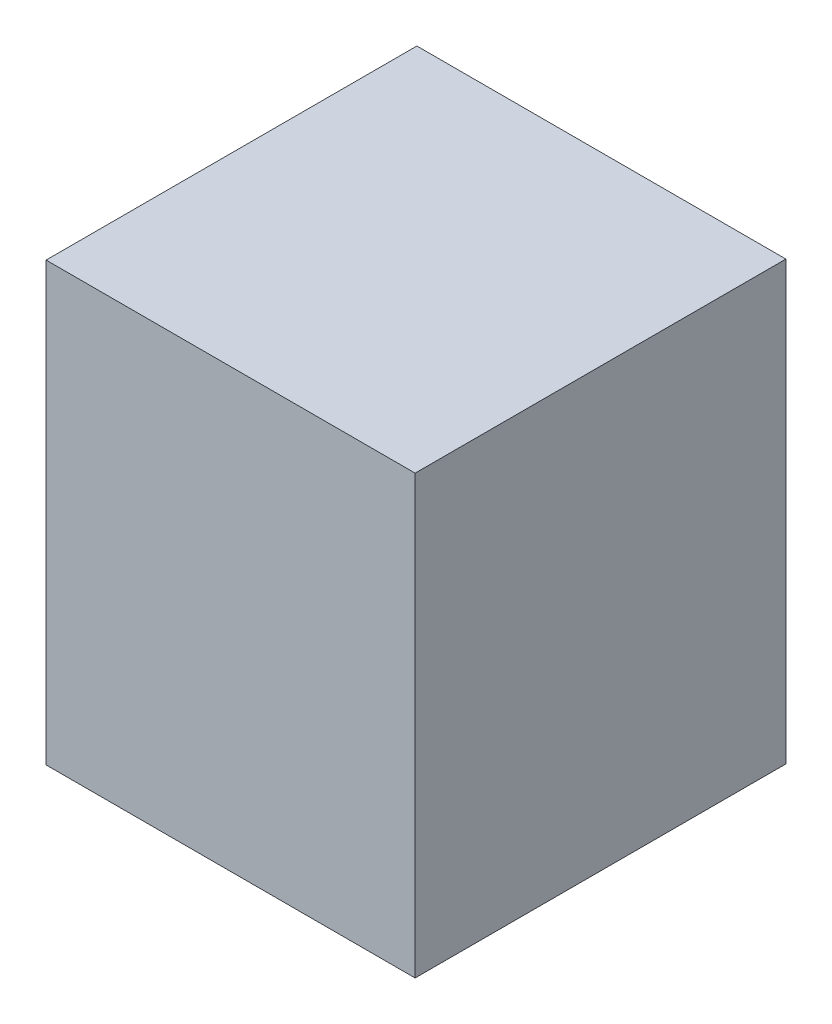
# Autodesk Inventor part: 3d printing workspace
Saved by Autodesk Inventor 2021 (Build 250183000, 183)
## iProperties
Created: 2021-11-22
Part Number: 3d printing workspace
Material: Generic
Document SubType Name: Sheet Metal
Designer: techv
Mass: 11183 g
Surface Area: 3009.64 cm^2
Volume: 11183 cm^3
Density: 1 g/cm^3
Sheet Metal Rule: Default
Appearance: Default
Author: techv
Autodesk Inventor part; units mm, degrees
ref_plane "YZ Plane" through (0, 0, 0) normal (1, 0, 0) x (0, 1, 0)
ref_plane "XZ Plane" through (0, 0, 0) normal (0, 1, 0) x (-1, 0, 0)
ref_plane "XY Plane" through (0, 0, 0) normal (0, 0, 1) x (1, 0, 0)
sketch "Sketch1" plane through (0, 0, 0) normal (0, 1, 0) x (-1, 0, 0)
  line L0 (-105.5, 106) -> (105.5, 106)
  line L1 (105.5, 106) -> (105.5, -106)
  line L2 (105.5, -106) -> (-105.5, -106)
  line L3 (-105.5, -106) -> (-105.5, 106)
  line L4 (-105.5, 106) -> (105.5, -106) construction
  line L5 (105.5, 106) -> (-105.5, -106) construction
  point P0 (0, 0)
  dimension "d0" = 211
  dimension "d1" = 212
  constraints: 12 end point, 2 midpoint, 2 parallel, 1 horizontal, 1 perpendicular
  measures "d0" distance of L1.end L2.end
  measures "d1" distance of L0.end L1.end
extrude "Extrusion1" add sketch "Sketch1" along normal blind 250
equation "\"BendRadius\" = Thickness"
equation "\"BendReliefWidth\" = Thickness"
equation "\"BendReliefDepth\" = 0.5 * Thickness"
equation "\"CornerReliefSize\" = 4 * Thickness"
equation "\"MinimumRemnant\" = 2 * Thickness"
equation "\"TransitionRadius\" = BendRadius"
equation "\"JacobiRadiusSize\" = Thickness"
equation "\"GapSize\" = Thickness"
equation "\"Thickness\" = 0.5"
body "Solid1"
